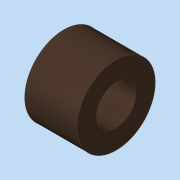
# Autodesk Inventor part: SleeveBearing3mm
Saved by Autodesk Inventor 2017 (Build 210142000, 142)
## iProperties
Created: 2016-12-01
Part Number: SleeveBearing3mm
Material: Bronze, Cast
Document SubType Name: Modeling
Designer: techn
Density: 8.87 g/cm^3
Appearance: Bronze - Satin
Author: techn
Autodesk Inventor part; units mm, degrees
ref_plane "YZ Plane" through (0, 0, 0) normal (1, 0, 0) x (0, 1, 0)
ref_plane "XZ Plane" through (0, 0, 0) normal (0, 1, 0) x (-1, 0, 0)
ref_plane "XY Plane" through (0, 0, 0) normal (0, 0, 1) x (1, 0, 0)
sketch "Sketch1" plane through (0, 0, 0) normal (0, 0, 1) x (1, 0, 0)
  line L0 (0, 0) -> (0, 1.5)
  line L1 (0, 0) -> (0, 3)
  line L2 (0, 3) -> (4, 3)
  line L3 (4, 3) -> (4, 1.5)
  line L4 (4, 1.5) -> (0, 1.5)
  line L5 (0, 0) -> (-3.024, 0)
  line L6 (0, 3) -> (4, 3)
  line L7 (4, 3) -> (4, 1.5)
  line L8 (4, 1.5) -> (0, 1.5)
  line L9 (0, 1.5) -> (0, 3)
  dimension "d0" = 1.5
  dimension "d1" = 3
  dimension "d2" = 4
  constraints: 20 end point, 3 horizontal, 3 perpendicular, 2 parallel, 2 vertical
  measures "d0" distance of L0.start L0.end
  measures "d1" distance of L0.start L1.end
  measures "d2" distance of L1.end L2.end
revolve "Revolution1" add sketch "Sketch1" angle 360 about axis through (0, 0, 0) along (-1, 0, 0)
body "Solid1"
